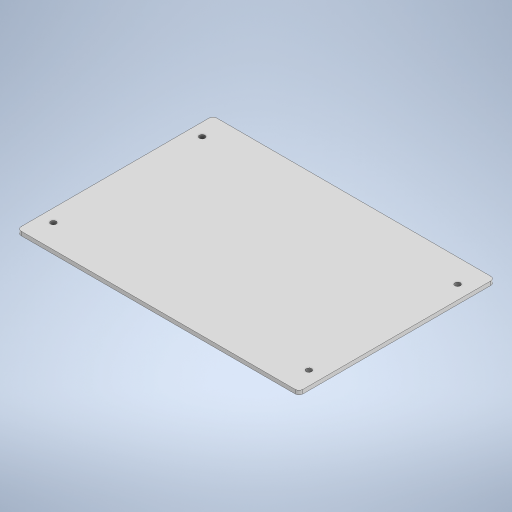
# Autodesk Inventor part: 뚜껑
Saved by Autodesk Inventor 2023 (Build 270158000, 158)
## iProperties
Created: 2023-08-30
Part Number: 뚜껑
Material: 일반
Document SubType Name: Modeling
Designer: rlatk
Density: 1 g/cm^3
Appearance: 기본값
Author: rlatk
Autodesk Inventor part; units mm, degrees
ref_plane "YZ Plane" through (0, 0, 0) normal (1, 0, 0) x (0, 1, 0)
ref_plane "XZ Plane" through (0, 0, 0) normal (0, 1, 0) x (-1, 0, 0)
ref_plane "XY Plane" through (0, 0, 0) normal (0, 0, 1) x (1, 0, 0)
sketch "스케치1" plane through (0, 0, 0) normal (0, 1, 0) x (-1, 0, 0)
  line L0 (72, -50) -> (-72, -50)
  line L1 (-72, -50) -> (-72, 50)
  line L2 (-72, 50) -> (72, 50)
  line L3 (72, 50) -> (72, -50)
  line L4 (72, -50) -> (-72, 50) construction
  line L5 (-72, -50) -> (72, 50) construction
  point P0 (0, 0)
  dimension "d0" = 144
  dimension "d1" = 100
  constraints: 12 end point, 2 midpoint, 2 parallel, 1 horizontal, 1 perpendicular
  measures "d0" distance of L1.end L2.end
  measures "d1" distance of L0.end L1.end
extrude "돌출1" add sketch "스케치1" along normal blind 2
fillet "모깎기1" radius 2 4 edges at (-72, 1, -50) (-72, 1, 50) (72, 1, 50) (72, 1, -50)
sketch "스케치2" plane through (0, 2, 0) normal (0, 1, 0) x (1, 0, 0)
  line L0 (72, -48) -> (72, 48) projected
  line L1 (70, 50) -> (-70, 50) projected
  line L2 (-72, 48) -> (-72, -48) projected
  line L3 (-72, 0) -> (72, 0)
  line L4 (-70, -50) -> (70, -50) projected
  line L5 (0, -50) -> (0, 50)
  point P0 (0, 0)
  point P1 (65, 38)
  point P2 (65, -38)
  point P3 (-65.5, 38)
  point P4 (-65.5, -38)
  dimension "d5" = 7
  dimension "d6" = 12
  dimension "d7" = 6.5
  dimension "d8" = 6.5
  dimension "d9" = 12
  dimension "d10" = 12
  constraints: 4 end point, 4 midpoint, 1 symmetric about line
  measures "d5" distance from line of L0 point (65, 38)
  measures "d6" distance from line of L1 point (65, 38)
  measures "d7" distance from line of L2 point (-65.5, 38)
  measures "d8" distance from line of L2 point (-65.5, -38)
  measures "d9" distance from line of L1 point (-65.5, 38)
  measures "d10" distance from line of L4 point (-65.5, -38)
hole "구멍1" at (65, 2, -38) at (65, 2, 38) at (-65.5, 2, -38) at (-65.5, 2, 38) direction (0, -1, 0) diameter 2.85 depth 10.4 tip angle 118 thread size "M3.5x0.6" class "6H" standard "ISO Metric profile"
